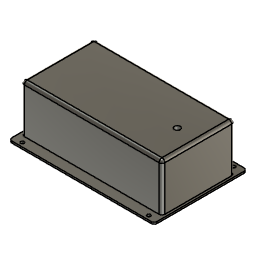
TR5_Modell_V1 (Autodesk Fusion 360 archive; units mm, degrees)
design "TR5_Modell_V1_Basis"
Autodesk Fusion 360 part; units mm, degrees
sketch "Skizze1" plane through (0, 0, 0) normal (0, 0, 1) x (1, 0, 0)
  line L0 (125, 0) -> (125, -80)
  line L1 (125, -80) -> (-125, -80)
  line L2 (-125, -80) -> (-125, 80)
  line L3 (-125, 80) -> (125, 80)
  line L4 (125, 80) -> (125, -80)
  line L5 (-125, 80) -> (-109, 80) construction
  line L6 (-109, 80) -> (-109, 76) construction
  circle A0 centre (-109, 73) radius 3 construction
  circle A1 centre (-109, 73) radius 3 construction
  circle A2 centre (-109, 73) radius 3
  line L7 (125, 80) -> (109, 80) construction
  line L8 (109, 80) -> (109, 76) construction
  circle A3 centre (109, 73) radius 3
  line L9 (-125, -80) -> (-109, -80) construction
  line L10 (-109, -80) -> (-109, -76) construction
  circle A4 centre (-109, -73) radius 3
  line L11 (125, -80) -> (109, -80) construction
  line L12 (109, -80) -> (109, -76) construction
  circle A5 centre (109, -73) radius 3
  dimension "d3" = 250
  dimension "d4" = 160
  dimension "d5" = 16
  dimension "d6" = 4
  dimension "d7" = 16
  dimension "d8" = 4
  dimension "d9" = 16
  dimension "d10" = 4
  dimension "d11" = 6
  dimension "d12" = 6
  dimension "d13" = 6
  dimension "d14" = 16
  dimension "d15" = 4
  dimension "d16" = 6
  constraint vertical L0
  constraint horizontal L1
  constraint vertical L2
  constraint horizontal L3
  constraint vertical L4
  constraint perpendicular L2 L5
  constraint perpendicular L3 L6
  constraint coincident L6.end A0
  constraint tangent A0 A1
  constraint coincident L6.end A1
  constraint tangent A1 A2
  constraint coincident L6.end A2
  constraint perpendicular L4 L7
  constraint perpendicular L3 L8
  constraint coincident L8.end A3
  constraint coincident L1 L9.end
  constraint perpendicular L9 L10
  constraint coincident L10.end A4
  constraint perpendicular L4 L11
  constraint perpendicular L1 L12
  constraint coincident L12.end A5
  measures "d3" distance of L0.end L1.end
  measures "d4" distance of L0.end L3.end
  measures "d5" distance of L2.end L5.end
  measures "d6" distance of L5.end L6.end
  measures "d7" distance of L3.end L7.end
  measures "d8" distance of L7.end L8.end
  measures "d9" distance of L1.end L9.end
  measures "d10" distance of L9.end L10.end
  measures "d11" diameter of A4
  measures "d12" diameter of A0
  measures "d13" diameter of A3
  measures "d14" distance of L0.end L11.end
  measures "d15" distance of L11.end L12.end
  measures "d16" diameter of A5
extrude "Extrusion1" add sketch "Skizze1" along normal blind 3
fillet "Abrundung1" radius 5 1 edges at (-125, -80, 1.5)
fillet "Abrundung2" radius 5 1 edges at (-125, 80, 1.5)
fillet "Abrundung3" radius 5 1 edges at (125, -80, 1.5)
fillet "Abrundung4" radius 5 1 edges at (125, 80, 1.5)
sketch "Skizze2" plane through (0, 0, 3) normal (0, 0, 1) x (-1, 0, 0)
  arc A0 (-125, -75) -> (-120, -80) centre (-120, -75) ccw
  line L0 (-120, -80) -> (120, -80)
  arc A1 (120, -80) -> (125, -75) centre (120, -75) ccw
  line L1 (125, -75) -> (125, 75)
  arc A2 (125, 75) -> (120, 80) centre (120, 75) ccw
  line L2 (120, 80) -> (-120, 80)
  arc A3 (-120, 80) -> (-125, 75) centre (-120, 75) ccw
  line L3 (-125, 75) -> (-125, -75)
  circle A4 centre (109, -73) radius 3
  circle A5 centre (109, 73) radius 3
  circle A6 centre (-109, -73) radius 3
  circle A7 centre (-109, 73) radius 3
  line L4 (0, 0) -> (121, 0) construction
  line L5 (0, 0) -> (-121, 0) construction
  line L6 (121, -62.5) -> (-121, -62.5)
  line L7 (-121, -62.5) -> (-121, 62.5)
  line L8 (-121, 62.5) -> (121, 62.5)
  line L9 (121, 62.5) -> (121, -62.5)
  line L10 (121, -62.5) -> (-121, 62.5) construction
  line L11 (-121, -62.5) -> (121, 62.5) construction
  dimension "d27" = 121
  dimension "d28" = 121
  dimension "d29" = 242
  dimension "d30" = 125
  constraint coincident L4.start L5.start
  constraint perpendicular L1 L4
  constraint parallel L4 L5
  constraint horizontal L6
  constraint perpendicular L6 L7
  constraint parallel L6 L8
  constraint parallel L7 L9
  constraint coincident L10 L4.start
  constraint coincident L11 L4.start
  measures "d27" distance of L4.start L4.end
  measures "d28" distance of L4.start L5.end
  measures "d29" distance of L7.end L8.end
  measures "d30" distance of L6.end L7.end
extrude "Extrusion2" add sketch "Skizze2" along normal blind 82 contours L6 L7 L8 L9
fillet "Abrundung5" radius 5 1 edges at (0, 62.5, 85)
fillet "Abrundung6" radius 5 1 edges at (0, -62.5, 85)
fillet "Abrundung7" radius 5 5 edges at (121, -62.5, 41.5) (121, -61.0355, 83.5355) (121, 0, 85) (121, 61.0355, 83.5355) (121, 62.5, 41.5)
fillet "Abrundung8" radius 5 5 edges at (-121, 62.5, 41.5) (-121, 61.0355, 83.5355) (-121, 0, 85) (-121, -61.0355, 83.5355) (-121, -62.5, 41.5)
sketch "Skizze4" plane through (0, 0, 85) normal (0, 0, 1) x (-1, 0, 0)
  line L0 (116, -57.5) -> (116, 57.5)
  line L1 (116, 57.5) -> (-116, 57.5)
  line L2 (-116, 57.5) -> (-116, -57.5)
  line L3 (-116, -57.5) -> (116, -57.5)
  line L4 (125, 0) -> (-85, 0) construction
  circle A0 centre (-85, 0) radius 5
  dimension "d43" = 210
  dimension "d44" = 10
  constraint horizontal L4
  constraint coincident L4.end A0.centre
  measures "d43" distance of L4.start L4.end
  measures "d44" diameter of A0
extrude "Extrusion3" cut sketch "Skizze4" against normal blind 10 contours A0
sketch "Skizze5" plane through (0, 0, 85) normal (0, 0, 1) x (-1, 0, 0)
  circle A0 centre (-85, 0) radius 5
  line L0 (116, -57.5) -> (116, 57.5)
  line L1 (116, 57.5) -> (-116, 57.5)
  line L2 (-116, 57.5) -> (-116, -57.5)
  line L3 (-116, -57.5) -> (116, -57.5)
extrude "Extrusion4" add sketch "Skizze5" against normal blind 35 contours A0
sketch "Skizze6" plane through (0, 0, 85) normal (0, 0, 1) x (-1, 0, 0)
  line L0 (116, -57.5) -> (116, 57.5)
  line L1 (116, 57.5) -> (-116, 57.5)
  line L2 (-116, 57.5) -> (-116, -57.5)
  line L3 (-116, -57.5) -> (116, -57.5)
  line L4 (125, 0) -> (-85, 0) construction
  circle A0 centre (-85, 0) radius 5
  dimension "d49" = 210
  dimension "d50" = 10
  constraint horizontal L4
  constraint coincident L4.end A0.centre
  measures "d49" distance of L4.start L4.end
  measures "d50" diameter of A0
extrude "Extrusion5" cut sketch "Skizze6" against normal blind 10 contours A0
